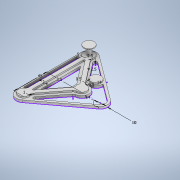
# Autodesk Inventor part: prot2
Saved by Autodesk Inventor 2022 (Build 260153000, 153)
## iProperties
Created: 2022-10-18
Part Number: prot2
Material: Genérico
Document SubType Name: Modeling
Designer: User
Density: 1 g/cm^3
Appearance: Valor por defecto
Author: User
Autodesk Inventor part; units mm, degrees
ref_plane "YZ Plane" through (0, 0, 0) normal (1, 0, 0) x (0, 1, 0)
ref_plane "XZ Plane" through (0, 0, 0) normal (0, 1, 0) x (-1, 0, 0)
ref_plane "XY Plane" through (0, 0, 0) normal (0, 0, 1) x (1, 0, 0)
sketch "Boceto1" plane through (0, 0, 0) normal (0, 1, 0) x (-1, 0, 0)
  circle A0 centre (1.5044, -21.0374) radius 7
  line L0 (0, 0) -> (-30, 0) construction
  line L1 (0, 0) -> (35.019, 45) construction
  arc A1 (45.0717, 45) -> (29.0132, 53.0615) centre (35.019, 45) ccw
  arc A2 (28.1996, -43.444) -> (39.4639, -39.5994) centre (35.019, -45) ccw
  arc A3 (29.0141, -53.0621) -> (45.0717, -45) centre (35.019, -45) ccw
  line L2 (45.0717, 45) -> (45.0717, -45)
  line L3 (-31.4523, -8.0252) -> (29.0141, -53.0621)
  line L4 (-31.4532, 8.0139) -> (29.0132, 53.0615)
  circle A4 centre (35.019, -45) radius 2.5
  line L5 (35.019, 45) -> (35.019, -45) construction
  line L6 (0, 0) -> (35.019, -45) construction
  arc A5 (39.4623, 39.5898) -> (28.1951, 43.4351) centre (35.019, 45) ccw
  line L7 (37.5264, -35.4953) -> (37.5264, 35.4947)
  line L8 (32.5115, -34.8171) -> (32.5115, 34.8171)
  line L9 (4.23, 5.4356) -> (6.2005, 3.9021) construction
  line L10 (7.7468, 5.9499) -> (30.7228, 35.4318)
  line L11 (3.8646, 8.971) -> (27.2206, 39.0273)
  line L12 (7.7468, -5.9499) -> (30.7228, -35.4318)
  line L13 (3.8646, -8.971) -> (27.2206, -39.0273)
  arc A6 (32.5115, 34.8171) -> (30.7228, 35.4318) centre (31.5115, 34.8171) ccw
  arc A7 (30.7228, -35.4318) -> (32.5115, -34.8171) centre (31.5115, -34.8171) ccw
  arc A8 (27.2206, 39.0273) -> (28.1951, 43.4351) centre (23.063, 42.2581) ccw
  arc A9 (-0.1798, 6.8852) -> (3.8646, 8.971) centre (-0.4077, 12.2909) ccw
  arc A10 (7.7468, 5.9499) -> (6.7608, 1.532) centre (11.9166, 2.7002) ccw
  arc A11 (6.7608, -1.532) -> (7.7468, -5.9499) centre (11.9166, -2.7002) ccw
  arc A12 (3.8646, -8.971) -> (-0.1798, -6.8852) centre (-0.4077, -12.2909) ccw
  arc A13 (6.7608, -1.532) -> (6.7608, 1.532) centre (0, 0) ccw
  arc A14 (-0.1798, 6.8852) -> (-0.1798, -6.8852) centre (0, 0) ccw
  arc A15 (39.4623, 39.5898) -> (37.5264, 35.4947) centre (42.8256, 35.4947) ccw
  arc A16 (37.5264, -35.4953) -> (39.4639, -39.5994) centre (42.8417, -35.4953) ccw
  arc A17 (28.1996, -43.444) -> (27.2206, -39.0273) centre (23.0492, -42.2688) ccw
  arc A18 (-31.4532, 8.0139) -> (-31.4523, -8.0252) centre (-25.4789, -0.0053) ccw
  line L14 (29.0115, 27.5422) -> (29.0115, -27.5422)
  line L15 (29.0115, -27.5422) -> (10.5075, -3.7984)
  arc A19 (10.1743, -2.3054) -> (10.5075, -3.7984) centre (11.9166, -2.7002) ccw
  arc A20 (10.1743, -2.3054) -> (10.1743, 2.3054) centre (0, 0) ccw
  arc A21 (10.5075, 3.7984) -> (10.1743, 2.3054) centre (11.9166, 2.7002) ccw
  line L16 (10.5075, 3.7984) -> (29.0115, 27.5422)
  line L17 (39.5264, 35.8019) -> (39.5264, -35.8019)
  line L18 (40.8447, 38.0421) -> (40.8447, -38.1418) construction
  line L19 (21.3809, 43.6361) -> (-23.936, 9.8749)
  arc A22 (23.8235, 40.3575) -> (21.3809, 43.6361) centre (22.6022, 41.9968) ccw
  arc A23 (-1.3686, 9.7923) -> (-9.8875, 0) centre (0, 0) ccw
  line L20 (23.8235, 40.3575) -> (1.2488, 11.3067)
  arc A24 (-1.3686, 9.7923) -> (1.2488, 11.3067) centre (-1.9249, 13.773) ccw
  arc A25 (-29.6624, 5.6176) -> (-29.9588, -5.3847) centre (-25.486, 0) ccw
  line L21 (-23.936, 9.8749) -> (-29.6624, 5.6176)
  arc A26 (-9.8875, 0) -> (-1.8786, -9.7074) centre (0, 0) ccw
  line L22 (43.1749, 35.8019) -> (43.1749, -35.8019)
  arc A27 (43.1749, 35.8019) -> (39.5264, 35.8019) centre (41.3506, 35.8019) ccw
  arc A28 (39.5264, -35.8019) -> (43.1749, -35.8019) centre (41.3506, -35.8019) ccw
  line L23 (-30, -5.3501) -> (-8.2939, -21.5174)
  arc A29 (2.552, -11.1194) -> (-1.8786, -9.7074) centre (-5.6513, -29.2032) ccw
  arc A30 (2.3012, -12.0728) -> (2.552, -11.1194) centre (2.3454, -11.5747) ccw
  arc A31 (-8.2939, -21.5174) -> (-7.4953, -21.1122) centre (-7.9953, -21.1164) ccw
  line L24 (11.2288, -22.5221) -> (24.908, -40.1255)
  line L25 (3.8504, -30.5629) -> (21.4406, -43.6644)
  arc A32 (21.4406, -43.6644) -> (24.908, -40.1255) centre (22.9339, -41.6595) ccw
  arc A33 (2.3012, -12.0728) -> (-2.6092, -13.0325) centre (1.5044, -21.0374) ccw
  arc A34 (-5.1216, -14.9468) -> (-7.4953, -21.1122) centre (1.5044, -21.0374) ccw
  arc A35 (2.3012, -12.0728) -> (-7.4953, -21.1122) centre (1.5044, -21.0374) ccw
  arc A36 (4.0099, -29.6816) -> (10.3429, -22.7346) centre (1.5044, -21.0374) ccw
  arc A37 (11.2288, -22.5221) -> (10.3429, -22.7346) centre (10.834, -22.8289) ccw
  arc A38 (4.0099, -29.6816) -> (3.8504, -30.5629) centre (4.1491, -30.1619) ccw
  point P0 (31.1449, 35.9734)
  point P1 (32.5115, 35.4947)
  point P2 (32.5115, -35.4953)
  point P3 (32.5115, 35.4947)
  point P4 (31.1449, -35.9734)
  point P5 (-3.2933, -26.1347)
  point P6 (8.3262, -19.468)
  point P7 (-7.4247, -22.1648)
  point P8 (10.4887, -21.5697)
  point P9 (2.9812, -29.9154)
  point P10 (-2.6092, -13.0325)
  dimension "d0" = 14
  dimension "d1" = 45
  dimension "d2" = 5
  dimension "d3" = 1
  dimension "d4" = 10
  dimension "d5" = 3.5
  dimension "d6" = 2
  dimension "d7" = 3
  dimension "d8" = 14
  dimension "d20" = 0.5
  dimension "d23" = 2.5
  dimension "d24" = 2.5
  dimension "d25" = 0.5
  constraints: 82 point on circle, 52 end point, 39 centre point, 38 tangent, 13 point on line, 13 symmetric about line, 7 coincident, 5 parallel, 3 equal radius, 2 vertical, 1 perpendicular, 7 other
  measures "d0" diameter of A0
  measures "d1" distance from line of L0 L1.end
  measures "d2" diameter of A4
  measures "d3" radius of A6
  measures "d4" radius of A18
  measures "d5" distance between parallel lines of L8 L14
  measures "d6" distance between parallel lines of L7 L17
  measures "d7" radial gap between concentric circles of A23 A14
  measures "d8" diameter of A25
  measures "d20" radius of A30
  measures "d23" distance between parallel lines of L13 L24
  measures "d24" radius of A32
  measures "d25" radius of A37
extrude "Extrusión2" add sketch "Boceto1" along normal blind 5 contours A0 | A17 L13 A12 A14 A9 L11 A8 A5 A15 L7 A16 A2
extrude "Extrusión3" add sketch "Boceto1" along normal blind 15 contours A4
extrude "Extrusión4" add sketch "Boceto1" along normal blind 3 contours L2 A3 L3 A18 L4 A1
extrude "Extrusión5" add sketch "Boceto1" along normal blind 3 contours A7 L12 A11 A13 A10 L10 A6 L8
sketch "Boceto2" plane through (-35.019, 15, -45) normal (0, 1, 0) x (1, 0, 0)
  circle A0 centre (0, 0) radius 7
  point P0 (35.019, -45)
  dimension "d30" = 14
  constraints: 1 centre point
  measures "d30" diameter of A0
extrude "Extrusión6" add sketch "Boceto2" along normal blind 2
fillet "Empalme1" radius 2 1 edges at (-32.519, 15, -45)
fillet "Empalme2" radius 1 1 edges at (-42.019, 15, -45)
